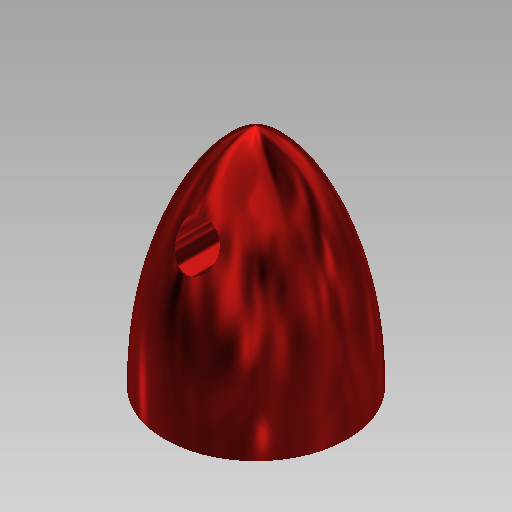
# Autodesk Inventor part: nose-over
Saved by Autodesk Inventor 2018.1 (Build 221171000, 171)
## iProperties
Created: 2013-08-26
Part Number: nose-over
Material: Generic
Document SubType Name: Modeling
Designer: Konstantin
Density: 1 g/cm^3
Appearance: Default
Mass: 3.10183 g
Surface Area: 15.6478 cm^2
Volume: 3.10183 cm^3
Author: Konstantin
Autodesk Inventor part; units mm, degrees
ref_plane "YZ Plane" through (0, 0, 0) normal (1, 0, 0) x (0, 1, 0)
ref_plane "XZ Plane" through (0, 0, 0) normal (0, 1, 0) x (-1, 0, 0)
ref_plane "XY Plane" through (0, 0, 0) normal (0, 0, 1) x (1, 0, 0)
sketch "Sketch1" plane through (0, 0, 0) normal (0, 0, 1) x (1, 0, 0)
  line L0 (0, 0) -> (0, 22.3)
  line L1 (0, 0) -> (9, 0)
  spline S0 degree 4 poles (0, 22.3) (5.9332, 19.4872) (8.095, 9.9218) (8.9717, 6.9333) (9, 0) knots 0 0 0 0 0 1 1 1 1 1
  point P0 (7.5, 11.15)
  point P1 (4.8515, 17.3878)
  point P2 (8.6406, 5.8553)
  constraints: 4 end point, 1 perpendicular, 1 vertical, 10 other
revolve "Revolution1" add sketch "Sketch1" angle 360 about axis through (0, 0, 0) along (0, 1, 0)
sketch "Sketch2" plane through (0, 0, 0) normal (0, 0, 1) x (1, 0, 0)
  circle A0 centre (0, 15) radius 2
  constraints: 1 centre point, 1 other
extrude "Extrusion1" cut sketch "Sketch2" along normal mid plane 15
sketch "Sketch3" plane through (0, 0, 0) normal (0, -1, 0) x (1, 0, 0)
  circle A0 centre (0, 0) radius 2.5
  dimension "d8" = 5
  constraints: 1 centre point, 1 coincident
  measures "d8" diameter of A0
extrude "Extrusion3" cut sketch "Sketch3" against normal blind 13
chamfer "Chamfer1" distance 0.5 angle 45 1 edges at (-2.5, 0, 0)
thread "Thread6" size "M5x0.8" class "6H" standard "ISO Metric profile" length 10
body "Solid1"
